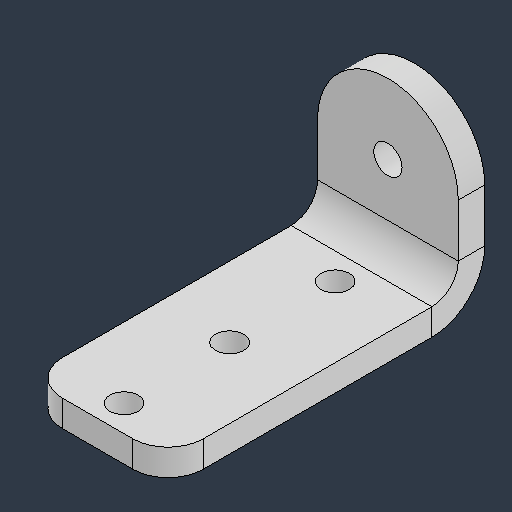
# Autodesk Inventor part: MOUNT,KICKER
Saved by Autodesk Inventor 2026 (Build 300175050, 175E)
## iProperties
Created: 2026-04-12
Part Number: MOUNT,KICKER
Material: Generic
Document SubType Name: Sheet Metal
Designer: Jthib
Mass: 9.00491 g
Surface Area: 50.2339 cm^2
Volume: 9.00491 cm^3
Density: 1 g/cm^3
Sheet Metal Rule: Default
Appearance: Default
Flat Pattern Width: 2.54 cm
Flat Pattern Length: 8.06225 cm
Flat Pattern Area: 20.4781 cm^2
Sheet Metal Width: 1.000 in
Sheet Metal Length: 3.174 in
Sheet Metal Area: 3.174 in^2
Author: Jthib
Autodesk Inventor part; units mm, degrees
ref_plane "YZ Plane" through (0, 0, 0) normal (1, 0, 0) x (0, 1, 0)
ref_plane "XZ Plane" through (0, 0, 0) normal (0, 1, 0) x (-1, 0, 0)
ref_plane "XY Plane" through (0, 0, 0) normal (0, 0, 1) x (1, 0, 0)
sketch "Sketch1" plane through (0, 0, 0) normal (0, 0, 1) x (1, 0, 0)
  line L0 (-17.78, 0) -> (17.78, 0) construction
  line L1 (-12.7, 0) -> (12.7, 0)
  line L2 (12.7, 0) -> (12.7, 19.05)
  arc A0 (12.7, 19.05) -> (-12.7, 19.05) centre (0, 19.05) ccw
  line L3 (-12.7, 19.05) -> (-12.7, 0)
  point P0 (0, 0)
  dimension "d0" = 25.4
  dimension "d1" = 19.05
  measures "d0" distance between parallel lines of L2 L3
  measures "d1" distance of L1.end L2.end
extrude "Plate1" add sketch "Sketch1" against normal blind 4.7625
sketch "Sketch2" plane through (12.7, 4.7625, -4.7625) normal (0, -1, 0) x (1, 0, 0)
  line L0 (-25.4, 0) -> (0, 0)
  line L1 (0, 0) -> (0, 57.15)
  line L2 (0, 57.15) -> (-25.4, 57.15)
  line L3 (-25.4, 57.15) -> (-25.4, 0)
  constraints: 6 end point, 1 horizontal, 1 perpendicular, 1 vertical
edge flange "Flange1" height 57.15 angle 90 thickness 4.7625 bend radius 4.7625 thickness toward (0, -1, 0) relief tear relief width 4.7625 relief depth 2.3813 edges at (0, 0, 0) wall of the first edge with corners at (-12.7, 4.7625, -4.7625) (12.7, 4.7625, -4.7625) (12.7, 4.7625, 52.3875) (-12.7, 4.7625, 52.3875)
bend "Bend1"
corner "Corner1"
sketch "Sketch3" plane through (0, 0, -4.7625) normal (0, 0, -1) x (-1, 0, 0)
  arc A0 (12.7, 19.05) -> (-12.7, 19.05) centre (0, 19.05) ccw construction
  point P0 (0, 0)
  constraints: 1 coincident
hole "Hole1" at (0, 19.05, -4.7625) direction (0, 0, 1) diameter 5.1054 end through all clearance for "Flat Head Machine Screw (82)" size "#10" standard "Ansi Unified Screw Threads"
sketch "Sketch4" plane through (-12.7, 4.7625, 52.3875) normal (0, 1, 0) x (1, 0, 0)
  line L0 (25.4, 47.625) -> (0, 47.625) construction
  line L1 (0, 47.625) -> (0, 0) construction
  line L2 (0, 0) -> (25.4, 0) construction
  line L3 (25.4, 47.625) -> (25.4, 0) construction
  line L4 (0, 0) -> (25.4, 47.625) construction
  line L5 (12.7, 4.7625) -> (12.7, 42.8625) construction
  point P0 (12.7, 52.3875)
  point P1 (12.7, 23.8125)
  dimension "d22" = 38.1
  constraints: 4 end point, 2 midpoint, 1 vertical
  measures "d22" distance of L5.start L5.end
hole "Hole2" at (0, 4.7625, 47.625) at (0, 4.7625, 28.575) at (0, 4.7625, 9.525) direction (0, -1, 0) diameter 5.1054 end through all clearance for "Flat Head Machine Screw (82)" size "#10" standard "Ansi Unified Screw Threads"
fillet "Corner Round1" radius 6.35 2 edges at (-12.7, 2.3812, 52.3875) (12.7, 2.3812, 52.3875)
equation "\"d20\" = Thickness"
equation "\"d4\" = Thickness"
equation "\"d5\" = BendReliefWidth"
equation "\"d6\" = BendReliefDepth"
equation "\"d7\" = MinimumRemnant"
equation "\"d8\" = TransitionRadius"
equation "\"d11\" = BendRadius"
equation "\"d12\" = CornerReliefSize"
equation "\"d13\" = GapSize"
equation "\"d14\" = JacobiRadiusSize"
equation "\"BendRadius\" = Thickness"
equation "\"BendReliefWidth\" = Thickness"
equation "\"BendReliefDepth\" = 0.5 * Thickness"
equation "\"CornerReliefSize\" = 4 * Thickness"
equation "\"MinimumRemnant\" = 2 * Thickness"
equation "\"TransitionRadius\" = BendRadius"
equation "\"JacobiRadiusSize\" = BendRadius"
equation "\"GapSize\" = Thickness"
equation "\"Thickness\" = 4.7625"
body "Solid2"
